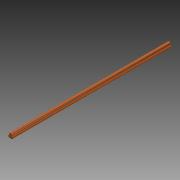
# Autodesk Inventor part: Front Railing
Saved by Autodesk Inventor 2015 (Build 190159000, 159)
## iProperties
Created: 2014-05-27
Part Number: Front Railing
Material: Wood (Cherry)
Document SubType Name: Modeling
Designer: Haden
Density: 0.63 g/cm^3
Appearance: Cherry - Natural Low Gloss
Author: Haden
Autodesk Inventor part; units mm, degrees
ref_plane "YZ Plane" through (0, 0, 0) normal (1, 0, 0) x (0, 1, 0)
ref_plane "XZ Plane" through (0, 0, 0) normal (0, 1, 0) x (-1, 0, 0)
ref_plane "XY Plane" through (0, 0, 0) normal (0, 0, 1) x (1, 0, 0)
sketch "Sketch1" plane through (0, 0, 0) normal (0, 0, 1) x (1, 0, 0)
  line L0 (0, 0) -> (25.4, 0) construction
  line L1 (0, 38.1) -> (15.24, 38.1) construction
  line L2 (0, 25.4) -> (12.7, 25.4) construction
  line L3 (0, 44.45) -> (2.54, 44.45)
  line L4 (0, -6.35) -> (2.54, -6.35)
  line L5 (0, 12.7) -> (25.4, 12.7) construction
  line L6 (0, 44.45) -> (0, -6.35) construction
  spline S0 degree 4 poles (2.54, 44.45) (5.3009, 44.45) (10.9391, 44.45) (21.7712, 35.5711) (3.7349, 22.5729) (30.1792, 15.4375) (30.3135, -1.1592) (14.7173, -6.35) (6.6645, -6.35) (2.54, -6.35) knots 0 0 0 0 0 0.138914 0.28369 0.472924 0.675915 0.83401 1 1 1 1 1
  line L7 (0, 44.45) -> (-2.54, 44.45)
  line L8 (0, -6.35) -> (-2.54, -6.35)
  spline S1 degree 4 poles (-2.54, 44.45) (-5.3009, 44.45) (-10.9391, 44.45) (-21.7712, 35.5711) (-3.7349, 22.5729) (-30.1792, 15.4375) (-30.3135, -1.1592) (-14.7173, -6.35) (-6.6645, -6.35) (-2.54, -6.35) knots 0 0 0 0 0 0.138914 0.28369 0.472924 0.675915 0.83401 1 1 1 1 1
  point P0 (-25.4, 0)
  point P1 (-15.24, 38.1)
  point P2 (-12.7, 25.4)
  point P3 (-25.4, 12.7)
  dimension "d0" = 25.4
  dimension "d2" = 15.24
  dimension "d3" = 12.7
  dimension "d9" = 2.54
  dimension "d10" = 2.54
  dimension "d11" = 25.4
  dimension "d13" = 6.35
  dimension "d14" = 12.7
  dimension "d15" = 12.7
  dimension "d16" = 12.7
  dimension "d17" = 6.35
  constraints: 18 end point, 9 horizontal, 6 symmetric about line, 4 point on line, 1 perpendicular, 12 other
  measures "d0" distance of L0.start L0.end
  measures "d2" distance of L1.start L1.end
  measures "d3" distance of L2.start L2.end
  measures "d9" distance of L3.start L3.end
  measures "d10" distance of L4.start L4.end
  measures "d11" distance of L5.start L5.end
  measures "d13" distance between parallel lines of L0 L4
  measures "d14" distance between parallel lines of L5 L0
  measures "d15" distance between parallel lines of L2 L5
  measures "d16" distance between parallel lines of L1 L2
  measures "d17" distance between parallel lines of L3 L1
extrude "Extrusion1" add sketch "Sketch1" along normal blind 1778
body "Solid1"
